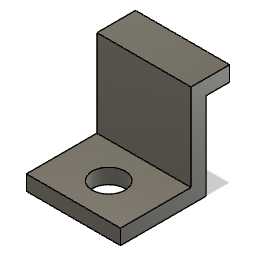
BreadboardClamp (Autodesk Fusion 360 design; units mm, degrees)
Autodesk Fusion 360 part; units mm, degrees
sketch "Sketch1" plane through (0, 0, 0) normal (0, 1, 0) x (1, 0, 0)
  line L0 (0, 0) -> (10, 0)
  line L1 (10, 0) -> (10, -9.1)
  line L2 (10, -9.1) -> (0, -9.1)
  line L3 (0, -9.1) -> (0, 0)
  line L4 (0, 0) -> (10, 0)
  line L5 (10, 0) -> (10, -1.6)
  line L6 (10, -1.6) -> (0, -1.6)
  line L7 (0, -1.6) -> (0, 0)
  point P0 (5, -5.35)
  dimension "d1" = 1.6
  dimension "d2" = 7.5
  dimension "d3" = 10
  dimension "d10" = 5
  dimension "d11" = 3.75
  constraint horizontal L0
  constraint vertical L1
  constraint horizontal L2
  constraint vertical L3
  constraint coincident L0.start L3.end
  constraint horizontal L4
  constraint vertical L5
  constraint horizontal L6
  constraint vertical L7
  constraint coincident L1 L5.end
  measures "d1" distance of L0 L6
  measures "d2" distance of L2 L6
  measures "d3" distance of L1.end L2.end
  measures "d10" distance of L1 P0
  measures "d11" distance of L2 P0
extrude "Extrude1" add sketch "Sketch1" against normal blind 1.6
extrude "Extrude2" add sketch "Sketch1" along normal blind 9.25 contours L0 L1 L3 L4 L5 L6 L7
sketch "Sketch2" plane through (0, 0, 0) normal (0, 0, -1) x (-1, 0, 0)
  line L0 (-10, 9.25) -> (-10, -1.6)
  line L1 (-10, -1.6) -> (0, -1.6)
  line L2 (0, -1.6) -> (0, 9.25)
  line L3 (0, 9.25) -> (-10, 9.25)
  line L4 (-10, 9.25) -> (0, 9.25)
  line L5 (0, 9.25) -> (0, 7.65)
  line L6 (0, 7.65) -> (-10, 7.65)
  line L7 (-10, 7.65) -> (-10, 9.25)
  dimension "d15" = 1.6
  constraint horizontal L4
  constraint vertical L5
  constraint horizontal L6
  constraint vertical L7
  constraint coincident L2 L5.end
  constraint coincident L0.start L3.end
  measures "d15" distance of L0.start L6.end
extrude "Extrude3" add sketch "Sketch2" along normal blind 2.5 contours L0 L2 L3 L4 L5 L6 L7
hole "Hole1" at (5, 0, 5.35) direction (0, -1, 0) diameter 3.5 depth 3 tip angle 118
equation "d10 = d3 / 2"
equation "d11 = d2 / 2"
